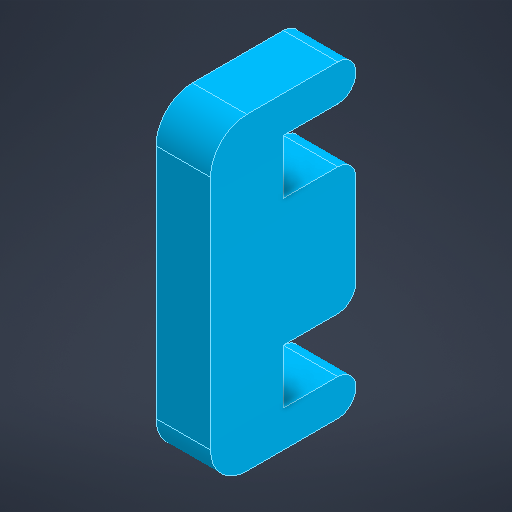
# Autodesk Inventor part: support
Saved by Autodesk Inventor 2025.3 (Build 293356030, 356C)
## iProperties
Created: 2025-09-05
Part Number: support
Material: 木材 (楓木)
Document SubType Name: Modeling
Designer: 陳泓任
Density: 0.67 g/cm^3
Appearance: 中天空藍
Author: 陳泓任
Autodesk Inventor part; units mm, degrees
ref_plane "YZ Plane" through (0, 0, 0) normal (1, 0, 0) x (0, 1, 0)
ref_plane "XZ Plane" through (0, 0, 0) normal (0, 1, 0) x (-1, 0, 0)
ref_plane "XY Plane" through (0, 0, 0) normal (0, 0, 1) x (1, 0, 0)
sketch "草圖1" plane through (0, 0, 0) normal (1, 0, 0) x (0, 1, 0)
  line L0 (-8.5, 0) -> (-8.5, -8)
  line L1 (-8.5, -8) -> (-6.5, -8)
  line L2 (-6.5, -8) -> (-6.5, -4)
  line L3 (-6.5, -4) -> (-3.5, -4)
  line L4 (3.5, -4) -> (3.5, -8)
  line L5 (3.5, -8) -> (-3.5, -8)
  line L6 (8.5, 0) -> (8.5, -8)
  line L7 (8.5, -8) -> (6.5, -8)
  line L8 (6.5, -8) -> (6.5, -4)
  line L9 (6.5, -4) -> (3.5, -4)
  line L10 (8.5, 0) -> (-8.5, 0)
  line L11 (-3.5, -8) -> (-3.5, -4)
  point P0 (0, 0)
  point P1 (0, 0)
  point P2 (0, 0)
  dimension "d2" = 3
  dimension "d3" = 7
  dimension "d4" = 8
  dimension "d5" = 4
  dimension "d6" = 2
  dimension "d12" = 17
  constraints: 24 end point, 7 perpendicular, 5 collinear, 2 coincident, 1 horizontal, 1 midpoint, 1 vertical
  measures "d2" distance of L2.end L3.end
  measures "d3" distance of L4.end L5.end
  measures "d4" distance of L6.start L6.end
  measures "d5" distance of L4.start L4.end
  measures "d6" distance of L6.end L7.end
  measures "d12" distance of L6.start L0.start
extrude "擠出1" add sketch "草圖1" along normal blind 3
fillet "圓角1" radius 2 2 edges at (1.5, 8.5, 0) (1.5, -8.5, 0)
fillet "圓角2" radius 1 4 edges at (1.5, 6.5, -8) (1.5, 3.5, -8) (1.5, -3.5, -8) (1.5, -6.5, -8)
fillet "圓角3" radius 1 2 edges at (1.5, 8.5, -8) (1.5, -8.5, -8)
